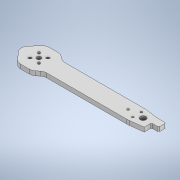
# Autodesk Inventor part: TokerCNC arm
Saved by Autodesk Inventor 2020 (Build 240168000, 168)
## iProperties
Created: 2022-08-18
Part Number: TokerCNC arm
Material: Generic
Document SubType Name: Modeling
Designer: Steven
Density: 1 g/cm^3
Appearance: Default
Author: Steven
Autodesk Inventor part; units mm, degrees
ref_plane "YZ Plane" through (0, 0, 0) normal (1, 0, 0) x (0, 1, 0)
ref_plane "XZ Plane" through (0, 0, 0) normal (0, 1, 0) x (-1, 0, 0)
ref_plane "XY Plane" through (0, 0, 0) normal (0, 0, 1) x (1, 0, 0)
sketch "Sketch1" plane through (0, 0, 0) normal (0, 1, 0) x (-1, 0, 0)
  arc A0 (-166.5, -1.5) -> (-165, 0) centre (-166.5, 0) ccw
  line L0 (-165, 0) -> (-158, 0)
  arc A1 (-158, 0) -> (-156.5, 1.5) centre (-158, 1.5) ccw
  line L1 (-156.5, 1.5) -> (-156.5, 10)
  line L2 (-156.5, 10) -> (-138.6622, 12.2297)
  arc A2 (-134.321, 12.5) -> (-138.6622, 12.2297) centre (-134.321, -22.5) ccw
  line L3 (-134.321, 12.5) -> (-23.3333, 12.5)
  arc A3 (-23.3333, 12.5) -> (-17.3333, 14.5) centre (-23.3333, 22.5) ccw
  line L4 (-17.3333, 14.5) -> (-12.6667, 18)
  arc A4 (-6.6667, 20) -> (-12.6667, 18) centre (-6.6667, 10) ccw
  line L5 (-6.6667, 20) -> (5.4953, 20)
  arc A5 (12.9849, 16.6262) -> (5.4953, 20) centre (5.4953, 10) ccw
  line L6 (12.9849, 16.6262) -> (21.8321, 6.6262)
  arc A6 (21.8321, -6.6262) -> (21.8321, 6.6262) centre (14.3426, 0) ccw
  line L7 (21.8321, -6.6262) -> (12.9849, -16.6262)
  arc A7 (5.4953, -20) -> (12.9849, -16.6262) centre (5.4953, -10) ccw
  line L8 (5.4953, -20) -> (-6.6667, -20)
  arc A8 (-12.6667, -18) -> (-6.6667, -20) centre (-6.6667, -10) ccw
  line L9 (-12.6667, -18) -> (-17.3333, -14.5)
  arc A9 (-17.3333, -14.5) -> (-23.3333, -12.5) centre (-23.3333, -22.5) ccw
  line L10 (-23.3333, -12.5) -> (-134.321, -12.5)
  arc A10 (-138.6622, -12.2297) -> (-134.321, -12.5) centre (-134.321, 22.5) ccw
  line L11 (-138.6622, -12.2297) -> (-156.5, -10)
  line L12 (-156.5, -10) -> (-165, -10)
  arc A11 (-166.5, -8.5) -> (-165, -10) centre (-165, -8.5) ccw
  line L13 (-166.5, -8.5) -> (-166.5, -1.5)
  arc A12 (4.5962, 6.7175) -> (6.7175, 4.5962) centre (5.6569, 5.6569) ccw
  line L14 (6.7175, 4.5962) -> (7.7782, 5.6569)
  arc A13 (7.7782, 5.6569) -> (5.6569, 7.7782) centre (6.7175, 6.7175) ccw
  line L15 (5.6569, 7.7782) -> (4.5962, 6.7175)
  line L16 (-4.5962, -6.7175) -> (-5.6569, -7.7782)
  arc A14 (-7.7782, -5.6569) -> (-5.6569, -7.7782) centre (-6.7175, -6.7175) ccw
  line L17 (-7.7782, -5.6569) -> (-6.7175, -4.5962)
  arc A15 (-4.5962, -6.7175) -> (-6.7175, -4.5962) centre (-5.6569, -5.6569) ccw
  arc A16 (6.7175, -4.5962) -> (4.5962, -6.7175) centre (5.6569, -5.6569) ccw
  line L18 (4.5962, -6.7175) -> (5.6569, -7.7782)
  arc A17 (5.6569, -7.7782) -> (7.7782, -5.6569) centre (6.7175, -6.7175) ccw
  line L19 (7.7782, -5.6569) -> (6.7175, -4.5962)
  line L20 (-5.6569, 7.7782) -> (-4.5962, 6.7175)
  arc A18 (-6.7175, 4.5962) -> (-4.5962, 6.7175) centre (-5.6569, 5.6569) ccw
  line L21 (-6.7175, 4.5962) -> (-7.7782, 5.6569)
  arc A19 (-5.6569, 7.7782) -> (-7.7782, 5.6569) centre (-6.7175, 6.7175) ccw
  circle A20 centre (-136.5, -6) radius 1.5
  circle A21 centre (-124.0736, 0) radius 1.5
  circle A22 centre (-144.9332, 0) radius 4
  circle A23 centre (0, 0) radius 3
  circle A24 centre (-136.5, 6) radius 1.5
  point P0 (5.4953, -20)
  point P1 (12.9849, -16.6262)
  point P2 (21.8321, -6.6262)
  point P3 (21.8321, 6.6262)
  point P4 (-12.6667, 18)
  point P5 (-165, -10)
  point P6 (7.7782, 5.6569)
  point P7 (5.6569, 7.7782)
  point P8 (6.7175, -4.5962)
  point P9 (5.6569, -7.7782)
  point P10 (4.5962, -6.7175)
  point P11 (-4.5962, -6.7175)
  point P12 (-5.6569, -7.7782)
  point P13 (-6.7175, -4.5962)
  point P14 (-7.7782, 5.6569)
  point P15 (-5.6569, 7.7782)
  constraints: 44 end point, 40 point on circle, 25 centre point
extrude "Extrusion1" add sketch "Sketch1" along normal blind 6
body "Solid1"
